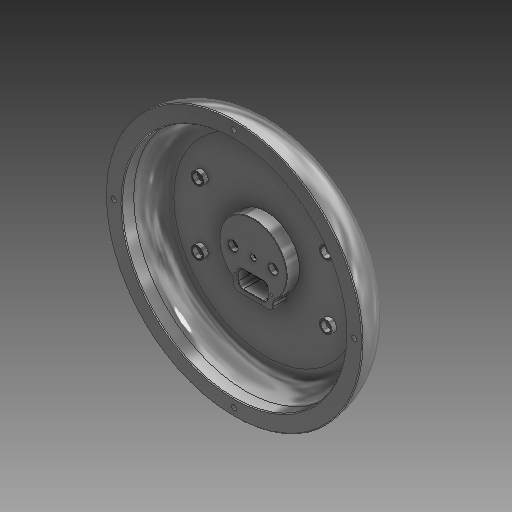
# Autodesk Inventor part: bottom cover
Saved by Autodesk Inventor 2019 (Build 230136000, 136)
## iProperties
Created: 2018-05-08
Part Number: bottom cover
Material: Aluminum 6061
Document SubType Name: Modeling
Designer: SimonD
Density: 2.7 g/cm^3
Appearance: Machined - Aluminum
Author: SimonD
Autodesk Inventor part; units mm, degrees
ref_plane "YZ Plane" through (0, 0, 0) normal (1, 0, 0) x (0, 1, 0)
ref_plane "XZ Plane" through (0, 0, 0) normal (0, 1, 0) x (-1, 0, 0)
ref_plane "XY Plane" through (0, 0, 0) normal (0, 0, 1) x (1, 0, 0)
sketch "Sketch1" plane through (0, 0, 0) normal (0, 0, 1) x (1, 0, 0)
  circle A0 centre (0, 0) radius 80
  dimension "d0" = 160
  constraints: 1 centre point, 1 coincident
  measures "d0" diameter of A0
extrude "Extrusion1" add sketch "Sketch1" along normal blind 27.5
sketch "Sketch2" plane through (0, 0, 27.5) normal (0, 0, 1) x (1, 0, 0)
  circle A0 centre (0, 0) radius 70
  dimension "d3" = 140
  constraints: 1 centre point, 1 coincident
  measures "d3" diameter of A0
extrude "Extrusion2" cut sketch "Sketch2" against normal blind 20
fillet "Fillet3" radius 12.5 1 edges at (-70, 0, 7.5)
fillet "Fillet4" radius 27.5 1 edges at (-80, 0, 0)
sketch "Sketch4" plane through (0, 0, 7.5) normal (0, 0, 1) x (1, 0, 0)
  circle A0 centre (0, 0) radius 21
  dimension "d13" = 42
  constraints: 1 centre point, 1 coincident
  measures "d13" diameter of A0
extrude "Extrusion4" add sketch "Sketch4" along normal blind 8
sketch "Sketch6" plane through (0, 0, 27.5) normal (0, 0, 1) x (1, 0, 0)
  point P0 (0, 0)
  point P1 (0, 75)
  point P2 (75, 0)
  point P3 (0, -75)
  point P4 (-75, 0)
  dimension "d24" = 75
  dimension "d25" = 75
  dimension "d26" = 75
  measures "d24" distance of point (75, 0) point (0, 0)
  measures "d25" distance of point (0, 0) point (0, 75)
  measures "d26" distance of point (0, -75) point (0, 0)
hole "Hole2" at (0, 75, 27.5) at (75, 0, 27.5) at (0, -75, 27.5) at (-75, 0, 27.5) direction (0, 0, -1) diameter 3.242 depth 10 thread size "M4x0.7" class "6H" standard "ISO Metric profile"
sketch "Sketch8" plane through (0, 0, 15.5) normal (0, 0, 1) x (1, 0, 0)
  point P0 (0, 0)
  point P1 (0, 0)
  constraints: 1 coincident
hole "Hole4" at (0, 0, 15.5) direction (0, 0, -1) diameter 3.5 end through all
sketch "Sketch9" plane through (0, 0, 0) normal (0, 0, -1) x (-1, 0, 0)
  circle A0 centre (0, 0) radius 1.75 projected
  circle A1 centre (0, 0) radius 19
  dimension "d56" = 38
  constraints: 1 centre point, 1 coincident
  measures "d56" diameter of A1
extrude "Extrusion5" cut sketch "Sketch9" against normal blind 9
sketch "Sketch10" plane through (0, 0, 9) normal (0, 0, -1) x (-1, 0, 0)
  circle A0 centre (0, 0) radius 1.75 projected
  circle A1 centre (0, 0) radius 6.75
  dimension "d59" = 13.5
  constraints: 1 centre point, 1 coincident
  measures "d59" diameter of A1
extrude "Extrusion6" cut sketch "Sketch10" against normal blind 4.6
sketch "Sketch11" plane through (0, 0, 15.5) normal (0, 0, 1) x (1, 0, 0)
  point P0 (0, 0)
  point P1 (12.5, 0)
  point P2 (-12.5, 0)
  dimension "d74" = 12.5
  dimension "d75" = 12.5
  measures "d74" distance of point (12.5, 0) point (0, 0)
  measures "d75" distance of point (-12.5, 0) point (0, 0)
hole "Hole5" at (12.5, 0, 15.5) at (-12.5, 0, 15.5) direction (0, 0, -1) diameter 3.2 end through all counterbore diameter 6 counterbore depth 3.2
sketch "Sketch13" plane through (0, 0, 7.5) normal (0, 0, 1) x (1, 0, 0)
  circle A0 centre (0, 0) radius 21 projected
  line L0 (12.5, -16.8745) -> (12.5, -23.249)
  line L1 (12.5, -23.249) -> (-12.5, -23.249)
  line L2 (-12.5, -23.249) -> (-12.5, -16.8745)
  dimension "d88" = 25
  dimension "d89" = 12.5
  constraints: 6 end point, 2 perpendicular, 2 point on circle, 1 vertical
  measures "d88" distance of L0.end L1.end
  measures "d89" distance from line of L0 point (0, 0)
extrude "Extrusion7" add sketch "Sketch13" along normal blind 8 contours A0 L0 L1 L2
sketch "Sketch18" plane through (0, 0, 15.5) normal (0, 0, 1) x (1, 0, 0)
  point P0 (0, 0)
  point P1 (11.3, -14.5)
  point P2 (-11.3, -14.5)
  dimension "d119" = 14.5
  dimension "d120" = 11.3
  dimension "d121" = 11.3
  dimension "d122" = 14.5
  measures "d119" vertical distance of point (11.3, -14.5) point (0, 0)
  measures "d120" horizontal distance of point (11.3, -14.5) point (0, 0)
  measures "d121" horizontal distance of point (-11.3, -14.5) point (0, 0)
  measures "d122" vertical distance of point (-11.3, -14.5) point (0, 0)
hole "Hole8" at (11.3, -14.5, 15.5) at (-11.3, -14.5, 15.5) direction (0, 0, -1) diameter 1.567 depth 5 thread size "M2x0.4" class "6H" standard "ISO Metric profile"
sketch "Sketch20" plane through (0, 0, 15.5) normal (0, 0, 1) x (1, 0, 0)
  line L0 (9.25, -9.249) -> (-9.25, -9.249)
  line L1 (-9.25, -9.249) -> (-9.25, -20.249)
  line L2 (-9.25, -20.249) -> (9.25, -20.249)
  line L3 (9.25, -20.249) -> (9.25, -9.249)
  line L4 (-12.5, -23.249) -> (12.5, -23.249) projected
  circle A0 centre (11.3, -14.5) radius 0.7835 projected
  point P0 (0, 0)
  dimension "d141" = 14
  dimension "d142" = 3
  dimension "d171" = 9.25
  dimension "d172" = 9.25
  constraints: 8 end point, 2 parallel, 1 horizontal, 1 perpendicular
  measures "d141" distance between parallel lines of L0 L4
  measures "d142" distance between parallel lines of L2 L4
  measures "d171" distance from line of L1 point (0, 0)
  measures "d172" distance from line of L3 point (0, 0)
extrude "Extrusion12" cut sketch "Sketch20" against normal blind 17 contours L3 L2 L1 L0
fillet "Fillet10" radius 3 4 edges at (9.25, -9.249, 12.25) (9.25, -20.249, 7.75) (-9.25, -9.249, 12.25) (-9.25, -20.249, 7.75)
fillet "Fillet11" radius 3 4 edges at (12.5, -16.8745, 11.5) (12.5, -23.249, 11.5) (-12.5, -23.249, 11.5) (-12.5, -16.8745, 11.5)
chamfer "Chamfer2" distance 0.25 angle 45 4 edges at (0, 21, 15.5) (-12.5, -19.2862, 15.5) (0, -23.249, 15.5) (12.5, -19.2862, 15.5)
sketch "Sketch21" plane through (0, 0, 7.5) normal (0, 0, 1) x (1, 0, 0)
  circle A0 centre (0, 0) radius 1.75 projected
  circle A1 centre (-40, -20) radius 4
  circle A2 centre (-40, 20) radius 4
  circle A3 centre (40, -20) radius 4
  circle A4 centre (40, 20) radius 4
  dimension "d147" = 40
  dimension "d148" = 20
  dimension "d149" = 20
  dimension "d150" = 20
  dimension "d151" = 20
  dimension "d152" = 40
  dimension "d153" = 40
  dimension "d154" = 40
  dimension "d155" = 8
  dimension "d156" = 8
  dimension "d157" = 8
  dimension "d158" = 8
  constraints: 4 centre point, 4 coincident
  measures "d147" horizontal distance of point (-40, -20) A0.centre
  measures "d148" vertical distance of point (-40, -20) point (0, 0)
  measures "d149" vertical distance of point (-40, 20) point (0, 0)
  measures "d150" vertical distance of point (40, -20) point (0, 0)
  measures "d151" vertical distance of point (40, 20) point (0, 0)
  measures "d152" horizontal distance of point (40, -20) point (0, 0)
  measures "d153" horizontal distance of point (40, 20) point (0, 0)
  measures "d154" horizontal distance of point (-40, 20) point (0, 0)
  measures "d155" diameter of A1
  measures "d156" diameter of A2
  measures "d157" diameter of A3
  measures "d158" diameter of A4
extrude "Extrusion13" add sketch "Sketch21" along normal blind 3 contours A1 | A2 | A3 | A4
sketch "Sketch22" plane through (-40, 20, 10.5) normal (0, 0, 1) x (1, 0, 0)
  circle A0 centre (0, -40) radius 4 projected
  circle A1 centre (80, 0) radius 4 projected
  circle A2 centre (80, -40) radius 4 projected
  point P0 (40, -20)
  point P1 (0, 0)
  constraints: 3 coincident
hole "Hole9" at (-40, -20, 10.5) at (-40, 20, 10.5) at (40, 20, 10.5) at (40, -20, 10.5) direction (0, 0, -1) diameter 3 end through all counterbore diameter 6 counterbore depth 3.2
chamfer "Chamfer3" distance 0.2 angle 45 19 edges at (36, -20, 10.5) (-44, -20, 10.5) (-44, 20, 10.5) (36, 20, 10.5) (-40, -17, 10.5) (40, -17, 10.5) (-40, 23, 10.5) (40, 23, 10.5) (8.3713, -10.1276, 15.5) (0, -9.249, 15.5) (-8.3713, -10.1276, 15.5) (-9.25, -14.749, 15.5) (-8.3713, -19.3703, 15.5) (0, -20.249, 15.5) (8.3713, -19.3703, 15.5) (9.25, -14.749, 15.5) (0, 1.75, 15.5) (-12.5, 3, 15.5) (12.5, 3, 15.5)
chamfer "Chamfer5" distance 1 angle 45 6 edges at (0, 19, 0) (0, -20.249, 0) (8.3713, -19.3703, 0) (9.25, -16.9226, 0) (-8.3713, -19.3703, 0) (-9.25, -16.9226, 0)
chamfer "Chamfer6" distance 0.5 angle 45 3 edges at (-70, 0, 27.5) (-80, 0, 27.4995) (-80, 0, 27.5)
body "Solid1"
